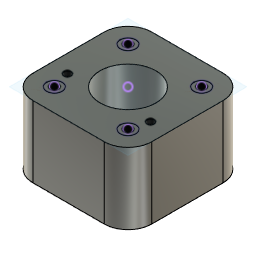
Z-Motor (Autodesk Fusion 360 design; units mm, degrees)
Autodesk Fusion 360 part; units mm, degrees
note: some values were not read from the file. Set by a fixed rule: which sketch regions a step uses.
sketch "Skizze1" plane through (0, 0, 0) normal (0, 0, 1) x (1, 0, 0)
  line L0 (0, 0) -> (50, 0)
  line L1 (50, 0) -> (50, 50)
  line L2 (50, 50) -> (0, 50)
  line L3 (0, 50) -> (0, 0)
  line L4 (25, 50) -> (25, -0.5033)
  circle A0 centre (25, 25) radius 11.75
  circle A1 centre (7.5, 17) radius 1.5
  circle A2 centre (42.5, 17) radius 1.5
  circle A3 centre (7.5, 25) radius 4.15
  circle A4 centre (42.5, 25) radius 4.15
  line L5 (9.5, 40.5) -> (40.5, 40.5)
  line L6 (40.5, 40.5) -> (40.5, 9.5)
  line L7 (40.5, 9.5) -> (9.5, 9.5)
  line L8 (9.5, 9.5) -> (9.5, 40.5)
  line L9 (0, 25) -> (50, 25)
  circle A5 centre (9.5, 40.5) radius 3.25
  circle A6 centre (40.5, 40.5) radius 3.25
  circle A7 centre (40.5, 9.5) radius 3.25
  circle A8 centre (9.5, 9.5) radius 3.25
  dimension "d1" = 50
  dimension "d2" = 50
  dimension "d3" = 23.5
  dimension "d4" = 3
  dimension "d5" = 3
  dimension "d6" = 35
  dimension "d7" = 17.5
  dimension "d8" = 8
  dimension "d9" = 8
  dimension "d10" = 25
  dimension "d11" = 8.3
  dimension "d12" = 8.3
  dimension "d13" = 25
  dimension "d14" = 25
  dimension "d15" = 17.5
  dimension "d16" = 17.5
  dimension "d29" = 31
  dimension "d30" = 31
  dimension "d31" = 15.5
  dimension "d32" = 15.5
  dimension "d33" = 6.5
  constraint horizontal L0
  constraint vertical L1
  constraint horizontal L2
  constraint vertical L3
  constraint coincident L0.start L3.end
  constraint midpoint L2 L4.start
  constraint perpendicular L0 L4
  constraint coincident L4 A0.centre
  constraint horizontal L5
  constraint vertical L6
  constraint horizontal L7
  constraint vertical L8
  constraint midpoint L3 L9.start
  constraint midpoint L1 L9.end
  constraint coincident L5.start L8.end
  constraint coincident L5.end L6.start
  constraint coincident L6.end L7.start
  constraint coincident L7.end L8.start
  constraint equal A5 A6
  constraint equal A6 A7
  constraint equal A7 A8
  measures "d1" distance of L0.start L2.end
  measures "d2" distance of L0.start L0.end
  measures "d3" diameter of A0
  measures "d4" diameter of A1
  measures "d5" diameter of A2
  measures "d6" horizontal distance of A1.centre A2.centre
  measures "d7" distance of L4 A1.centre
  measures "d8" vertical distance of A0.centre A1.centre
  measures "d9" vertical distance of A0.centre A2.centre
  measures "d10" distance of L2 A0.centre
  measures "d11" diameter of A3
  measures "d12" diameter of A4
  measures "d13" distance of L2 A3.centre
  measures "d14" distance of L2 A4.centre
  measures "d15" distance of L4 A3.centre
  measures "d16" distance of L4 A4.centre
  measures "d29" distance of L5.start L5.end
  measures "d30" distance of L5.start L7.end
  measures "d31" distance of L5 L9
  measures "d32" distance of L4 L8
  measures "d33" diameter of A5
extrude "Extrusion1" add sketch "Skizze1" along normal blind 30 contours L0 L3 L4 A3 L7 L8 L9 A8 | L0 L1 L4 A4 L6 L7 L9 A7 | L2 L3 L4 A3 L5 L8 L9 A5 | L4 A0 A3 L7 L8 L9 A8 | L4 A0 A4 L6 L7 L9 A7 | A3 L8 L9 | A3 L8 L9 | L1 L2 L4 A4 L5 L6 L9 A6 | L4 A0 A3 L5 L8 L9 A5 | A3 L8 L9 | A3 L8 L9 | A4 L6 L9 | A4 L6 L9 | L4 A0 A4 L5 L6 L9 A6 | A4 L6 L9 | A4 L6 L9 | A1 | A2
extrude "Extrusion2" cut sketch "Skizze1" along normal blind 20 contours A3 L8 L9 | A3 L8 L9 | A3 L8 L9 | A3 L8 L9 | A4 L6 L9 | A4 L6 L9 | A4 L6 L9 | A4 L6 L9
sketch "Skizze2" plane through (0, 0, 30) normal (0, 0, 1) x (-1, 0, 0)
  circle A0 centre (-25, -25) radius 11.75
  line L0 (0, -50) -> (0, 0)
  line L1 (0, 0) -> (-50, 0)
  line L2 (-50, 0) -> (-50, -50)
  line L3 (-50, -50) -> (0, -50)
  circle A1 centre (-7.5, -17) radius 1.5
  circle A2 centre (-42.5, -17) radius 1.5
  circle A3 centre (-40.5, -40.5) radius 3.25
  circle A4 centre (-9.5, -9.5) radius 3.25
  circle A5 centre (-40.5, -9.5) radius 3.25
  circle A6 centre (-9.5, -40.5) radius 3.25
  circle A7 centre (-9.5, -40.5) radius 3.25
  circle A8 centre (-40.5, -40.5) radius 3.25
  circle A9 centre (-40.5, -9.5) radius 3.25
  circle A10 centre (-9.5, -9.5) radius 3.25
  circle A11 centre (-9.5, -40.5) radius 1.75
  circle A12 centre (-40.5, -40.5) radius 1.75
  circle A13 centre (-40.5, -9.5) radius 1.75
  circle A14 centre (-9.5, -9.5) radius 1.75
  point P0 (-25, -25)
  dimension "d21" = 3
  dimension "d22" = 3
  dimension "d23" = 17.5
  dimension "d24" = 17.5
  dimension "d25" = 8
  dimension "d26" = 8
  dimension "d34" = 6.5
  dimension "d35" = 3.5
  constraint concentric A6 A7
  constraint concentric A3 A8
  constraint concentric A5 A9
  constraint concentric A4 A10
  constraint equal A7 A8
  constraint equal A7 A9
  constraint equal A7 A10
  constraint concentric A7 A11
  constraint concentric A3 A12
  constraint concentric A5 A13
  constraint concentric A4 A14
  constraint equal A11 A12
  constraint equal A11 A13
  constraint equal A11 A14
  measures "d21" diameter of A1
  measures "d22" diameter of A2
  measures "d23" horizontal distance of A2.centre P0
  measures "d24" horizontal distance of A1.centre P0
  measures "d25" vertical distance of A1.centre P0
  measures "d26" vertical distance of A2.centre P0
  measures "d34" diameter of A7
  measures "d35" diameter of A11
extrude "Extrusion3" cut sketch "Skizze2" against normal blind 15 contours A1 | A2
extrude "Extrusion4" add sketch "Skizze2" against normal blind 5 contours A3 A8 | A4 A10 | A5 A9 | A6 A7
fillet "Abrundung1" radius 10 4 edges at (50, 50, 15) (50, 0, 15) (0, 0, 15) (0, 50, 15)
equation "d7 = ( 35 / 2 ) * 1 mm"
equation "d31 = ( 31 / 2 ) * 1 mm"
equation "d32 = ( 31 / 2 ) * 1 mm"
